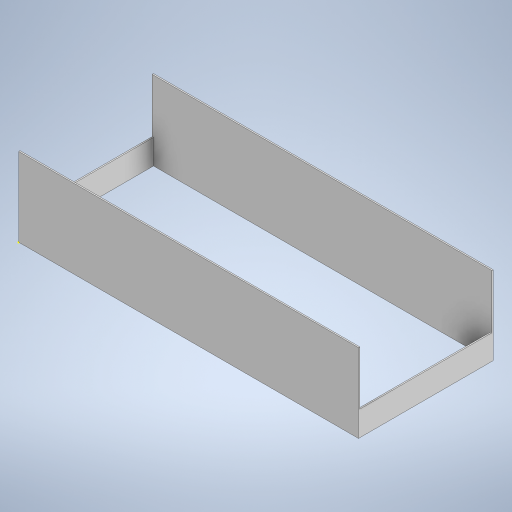
# Autodesk Inventor part: Walls
Saved by Autodesk Inventor 2023 (Build 270158030, 158C)
## iProperties
Created: 2024-02-01
Part Number: Walls
Material: Generic
Document SubType Name: Modeling
Designer: HP
Density: 1 g/cm^3
Appearance: Default
Author: HP
Autodesk Inventor part; units mm, degrees
ref_plane "YZ Plane" through (0, 0, 0) normal (1, 0, 0) x (0, 1, 0)
ref_plane "XZ Plane" through (0, 0, 0) normal (0, 1, 0) x (-1, 0, 0)
ref_plane "XY Plane" through (0, 0, 0) normal (0, 0, 1) x (1, 0, 0)
sketch "Sketch2" plane through (0, 0, 0) normal (1, 0, 0) x (0, 1, 0)
  line L0 (0, 0) -> (175, 0)
  line L1 (175, 0) -> (175, 3)
  line L2 (175, 3) -> (0, 3)
  line L3 (0, 3) -> (0, 0)
  line L4 (0, 300) -> (175, 300)
  line L5 (175, 300) -> (175, 297)
  line L6 (175, 297) -> (0, 297)
  line L7 (0, 297) -> (0, 300)
  dimension "d8" = 175
  dimension "d9" = 3
  dimension "d10" = 175
  dimension "d11" = 3
  constraints: 16 end point, 4 parallel, 2 horizontal, 2 perpendicular, 1 point on line
  measures "d8" distance of L2.end L1.end
  measures "d9" distance of L1.end L0.end
  measures "d10" distance of L5.end L6.end
  measures "d11" distance of L4.end L5.end
extrude "Extrusion2" add sketch "Sketch2" along normal blind 756
sketch "Sketch3" plane through (0, 0, 300) normal (0, 0, 1) x (1, 0, 0)
  point P0 (0, 0)
sketch "Sketch4" plane through (0, 0, 300) normal (0, 0, 1) x (1, 0, 0)
  line L0 (0, 0) -> (3, 0)
  line L1 (3, 0) -> (3, 55)
  line L2 (3, 55) -> (0, 55)
  line L3 (0, 55) -> (0, 0)
  line L4 (756, 0) -> (753, 0)
  line L5 (753, 0) -> (753, 55)
  line L6 (753, 55) -> (756, 55)
  line L7 (756, 55) -> (756, 0)
  dimension "d14" = 3
  dimension "d15" = 55
  dimension "d16" = 3
  dimension "d17" = 55
  constraints: 16 end point, 4 parallel, 2 horizontal, 2 perpendicular
  measures "d14" distance of L2.end L1.end
  measures "d15" distance of L1.end L0.end
  measures "d16" distance of L5.end L6.end
  measures "d17" distance of L4.end L5.end
extrude "Extrusion3" add sketch "Sketch4" against normal through all
sketch "Sketch5" plane through (0, 0, 300) normal (0, 0, 1) x (1, 0, 0)
  point P0 (0, 0)
body "Solid2"
